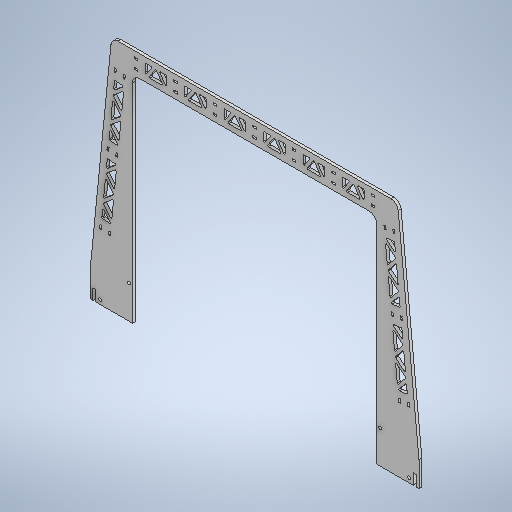
# Autodesk Inventor part: GateBrigeSideLessMaterial
Saved by Autodesk Inventor 2025.1 (Build 291241000, 241)
## iProperties
Created: 2025-03-30
Part Number: GateBrigeSideLessMaterial
Material: Všeobecné
Document SubType Name: Modeling
Designer: 42060
Density: 1 g/cm^3
Appearance: Výchozí
Author: 42060
Autodesk Inventor part; units mm, degrees
ref_plane "YZ Plane" through (0, 0, 0) normal (1, 0, 0) x (0, 1, 0)
ref_plane "XZ Plane" through (0, 0, 0) normal (0, 1, 0) x (-1, 0, 0)
ref_plane "XY Plane" through (0, 0, 0) normal (0, 0, 1) x (1, 0, 0)
sketch "Náčrt1" plane through (0, 0, 0) normal (0, 0, 1) x (1, 0, 0)
  line L0 (0, 0) -> (-160, 0)
  line L1 (-170, -10) -> (-170, -300)
  line L2 (-229, -300) -> (-229, -265.3)
  line L3 (-190.0509, 30) -> (0, 30)
  line L4 (0, 30) -> (0, 0)
  line L5 (-203.7, -249) -> (-170, -249)
  line L6 (-170, -249) -> (-170, -299)
  line L7 (-170, -299) -> (-220, -299)
  line L8 (-220, -299) -> (-220, -265.3)
  line L9 (-220, -265.3) -> (-203.7, -249)
  line L10 (-220, -299) -> (-170, -249) construction
  circle A0 centre (-215, -294) radius 2.1
  circle A1 centre (-175, -254) radius 2.1
  arc A2 (-160, 0) -> (-170, -10) centre (-160, -10) ccw
  line L11 (-200, 21.0077) -> (-229, -265.3)
  arc A3 (-190.0509, 30) -> (-200, 21.0077) centre (-190.0509, 20) ccw
  line L12 (-225, -300) -> (-225, -285)
  line L13 (-225, -285) -> (-221, -285)
  line L14 (-221, -285) -> (-221, -300)
  line L15 (-170, -300) -> (-221, -300)
  line L16 (-225, -300) -> (-229, -300)
  line L17 (0, 0) -> (160, 0)
  line L18 (170, -10) -> (170, -300)
  line L19 (229, -300) -> (229, -265.3)
  line L20 (190.0509, 30) -> (0, 30)
  line L21 (203.7, -249) -> (170, -249)
  line L22 (170, -249) -> (170, -299)
  line L23 (170, -299) -> (220, -299)
  line L24 (220, -299) -> (220, -265.3)
  line L25 (220, -265.3) -> (203.7, -249)
  line L26 (220, -299) -> (170, -249) construction
  circle A4 centre (215, -294) radius 2.1
  circle A5 centre (175, -254) radius 2.1
  arc A6 (170, -10) -> (160, 0) centre (160, -10) ccw
  line L27 (200, 21.0077) -> (229, -265.3)
  arc A7 (200, 21.0077) -> (190.0509, 30) centre (190.0509, 20) ccw
  line L28 (225, -300) -> (225, -285)
  line L29 (225, -285) -> (221, -285)
  line L30 (221, -285) -> (221, -300)
  line L31 (170, -300) -> (221, -300)
  line L32 (225, -300) -> (229, -300)
  line L33 (-36.6095, 9.0611) -> (-28.3278, 21.2788)
  line L34 (-26.6722, 21.2788) -> (-18.3905, 9.0611)
  line L35 (-19.2183, 7.5) -> (-35.7817, 7.5)
  line L36 (-21.6095, 20.9389) -> (-14.3278, 10.1964)
  line L37 (-12.5, 10.7575) -> (-12.5, 21.5)
  line L38 (-13.5, 22.5) -> (-20.7817, 22.5)
  line L39 (-33.3905, 20.9389) -> (-40.6722, 10.1964)
  line L40 (-42.5, 10.7575) -> (-42.5, 21.5)
  line L41 (-41.5, 22.5) -> (-34.2183, 22.5)
  line L42 (-55, 15) -> (0, 15) construction
  arc A8 (-41.5, 22.5) -> (-42.5, 21.5) centre (-41.5, 21.5) ccw
  arc A9 (-33.3905, 20.9389) -> (-34.2183, 22.5) centre (-34.2183, 21.5) ccw
  arc A10 (-42.5, 10.7575) -> (-40.6722, 10.1964) centre (-41.5, 10.7575) ccw
  arc A11 (-36.6095, 9.0611) -> (-35.7817, 7.5) centre (-35.7817, 8.5) ccw
  arc A12 (-19.2183, 7.5) -> (-18.3905, 9.0611) centre (-19.2183, 8.5) ccw
  arc A13 (-26.6722, 21.2788) -> (-28.3278, 21.2788) centre (-27.5, 20.7178) ccw
  arc A14 (-20.7817, 22.5) -> (-21.6095, 20.9389) centre (-20.7817, 21.5) ccw
  arc A15 (-12.5, 21.5) -> (-13.5, 22.5) centre (-13.5, 21.5) ccw
  arc A16 (-14.3278, 10.1964) -> (-12.5, 10.7575) centre (-13.5, 10.7575) ccw
  arc A17 (-81.6722, 21.2788) -> (-83.3278, 21.2788) centre (-82.5, 20.7178) ccw
  line L43 (-91.6095, 9.0611) -> (-83.3278, 21.2788)
  line L44 (-68.5, 22.5) -> (-75.7817, 22.5)
  arc A18 (-67.5, 21.5) -> (-68.5, 22.5) centre (-68.5, 21.5) ccw
  line L45 (-81.6722, 21.2788) -> (-73.3905, 9.0611)
  arc A19 (-74.2183, 7.5) -> (-73.3905, 9.0611) centre (-74.2183, 8.5) ccw
  line L46 (-76.6095, 20.9389) -> (-69.3278, 10.1964)
  line L47 (-74.2183, 7.5) -> (-90.7817, 7.5)
  arc A20 (-69.3278, 10.1964) -> (-67.5, 10.7575) centre (-68.5, 10.7575) ccw
  line L48 (-110, 15) -> (-55, 15) construction
  arc A21 (-96.5, 22.5) -> (-97.5, 21.5) centre (-96.5, 21.5) ccw
  arc A22 (-97.5, 10.7575) -> (-95.6722, 10.1964) centre (-96.5, 10.7575) ccw
  arc A23 (-91.6095, 9.0611) -> (-90.7817, 7.5) centre (-90.7817, 8.5) ccw
  arc A24 (-88.3905, 20.9389) -> (-89.2183, 22.5) centre (-89.2183, 21.5) ccw
  line L49 (-67.5, 10.7575) -> (-67.5, 21.5)
  arc A25 (-75.7817, 22.5) -> (-76.6095, 20.9389) centre (-75.7817, 21.5) ccw
  line L50 (-96.5, 22.5) -> (-89.2183, 22.5)
  line L51 (-88.3905, 20.9389) -> (-95.6722, 10.1964)
  line L52 (-97.5, 10.7575) -> (-97.5, 21.5)
  arc A26 (-136.6722, 21.2788) -> (-138.3278, 21.2788) centre (-137.5, 20.7178) ccw
  line L53 (-146.6095, 9.0611) -> (-138.3278, 21.2788)
  line L54 (-123.5, 22.5) -> (-130.7817, 22.5)
  arc A27 (-122.5, 21.5) -> (-123.5, 22.5) centre (-123.5, 21.5) ccw
  line L55 (-136.6722, 21.2788) -> (-128.3905, 9.0611)
  arc A28 (-129.2183, 7.5) -> (-128.3905, 9.0611) centre (-129.2183, 8.5) ccw
  line L56 (-131.6095, 20.9389) -> (-124.3278, 10.1964)
  line L57 (-129.2183, 7.5) -> (-145.7817, 7.5)
  arc A29 (-124.3278, 10.1964) -> (-122.5, 10.7575) centre (-123.5, 10.7575) ccw
  line L58 (-165, 15) -> (-110, 15) construction
  arc A30 (-151.5, 22.5) -> (-152.5, 21.5) centre (-151.5, 21.5) ccw
  arc A31 (-152.5, 10.7575) -> (-150.6722, 10.1964) centre (-151.5, 10.7575) ccw
  arc A32 (-146.6095, 9.0611) -> (-145.7817, 7.5) centre (-145.7817, 8.5) ccw
  arc A33 (-143.3905, 20.9389) -> (-144.2183, 22.5) centre (-144.2183, 21.5) ccw
  line L59 (-122.5, 10.7575) -> (-122.5, 21.5)
  arc A34 (-130.7817, 22.5) -> (-131.6095, 20.9389) centre (-130.7817, 21.5) ccw
  line L60 (-151.5, 22.5) -> (-144.2183, 22.5)
  line L61 (-143.3905, 20.9389) -> (-150.6722, 10.1964)
  line L62 (-152.5, 10.7575) -> (-152.5, 21.5)
  line L63 (-194.0109, -19.4488) -> (-184.1326, -20.4494)
  line L64 (-183.6011, -22.2191) -> (-194.48, -31.0969)
  line L65 (-196.1072, -30.2213) -> (-195.1066, -20.3429)
  line L66 (-182.544, -28.7227) -> (-184.7467, -50.4692)
  line L67 (-186.5164, -51.0007) -> (-196.2883, -39.0261)
  line L68 (-196.1458, -37.6191) -> (-184.1711, -27.8471)
  line L69 (-195.9642, -45.7498) -> (-186.1923, -57.7245)
  line L70 (-186.3348, -59.1315) -> (-198.3095, -68.9034)
  line L71 (-199.9366, -68.0279) -> (-197.7339, -46.2813)
  line L72 (-188.0006, -65.6537) -> (-199.9752, -75.4256)
  line L73 (-200.1177, -76.8326) -> (-190.3458, -88.8073)
  line L74 (-188.5761, -88.2758) -> (-186.3734, -66.5292)
  line L75 (-199.7937, -83.5564) -> (-190.9158, -94.4353)
  line L76 (-191.7914, -96.0625) -> (-201.6698, -95.0619)
  line L77 (-202.5639, -93.9662) -> (-201.5633, -84.0878)
  line L78 (-189.0718, -19.9491) -> (-188.1144, -10.4975) construction
  arc A35 (-194.0109, -19.4488) -> (-195.1066, -20.3429) centre (-194.1117, -20.4437) ccw
  arc A36 (-183.6011, -22.2191) -> (-184.1326, -20.4494) centre (-184.2333, -21.4443) ccw
  arc A37 (-196.1072, -30.2213) -> (-194.48, -31.0969) centre (-195.1123, -30.3221) ccw
  arc A38 (-196.1458, -37.6191) -> (-196.2883, -39.0261) centre (-195.5135, -38.3938) ccw
  arc A39 (-186.5164, -51.0007) -> (-184.7467, -50.4692) centre (-185.7416, -50.3685) ccw
  arc A40 (-182.544, -28.7227) -> (-184.1711, -27.8471) centre (-183.5389, -28.6219) ccw
  arc A41 (-195.9642, -45.7498) -> (-197.7339, -46.2813) centre (-196.739, -46.3821) ccw
  arc A42 (-186.3348, -59.1315) -> (-186.1923, -57.7245) centre (-186.9671, -58.3567) ccw
  arc A43 (-199.9366, -68.0279) -> (-198.3095, -68.9034) centre (-198.9417, -68.1287) ccw
  arc A44 (-199.9752, -75.4256) -> (-200.1177, -76.8326) centre (-199.343, -76.2004) ccw
  arc A45 (-190.3458, -88.8073) -> (-188.5761, -88.2758) centre (-189.571, -88.175) ccw
  arc A46 (-186.3734, -66.5292) -> (-188.0006, -65.6537) centre (-187.3683, -66.4284) ccw
  arc A47 (-199.7937, -83.5564) -> (-201.5633, -84.0878) centre (-200.5684, -84.1886) ccw
  arc A48 (-202.5639, -93.9662) -> (-201.6698, -95.0619) centre (-201.569, -94.067) ccw
  arc A49 (-191.7914, -96.0625) -> (-190.9158, -94.4353) centre (-191.6906, -95.0676) ccw
  arc A50 (-212.6413, -193.4572) -> (-211.7472, -194.5528) centre (-211.6464, -193.5579) ccw
  line L79 (-201.8688, -195.5534) -> (-211.7472, -194.5528)
  arc A51 (-201.8688, -195.5534) -> (-200.9932, -193.9263) centre (-201.768, -194.5585) ccw
  arc A52 (-200.4232, -188.2982) -> (-198.6535, -187.7667) centre (-199.6484, -187.666) ccw
  line L80 (-209.871, -183.0473) -> (-200.9932, -193.9263)
  line L81 (-212.6413, -193.4572) -> (-211.6407, -183.5788)
  arc A53 (-209.871, -183.0473) -> (-211.6407, -183.5788) centre (-210.6458, -183.6796) ccw
  line L82 (-198.078, -165.1446) -> (-210.0526, -174.9165)
  line L83 (-210.1951, -176.3236) -> (-200.4232, -188.2982)
  line L84 (-198.6535, -187.7667) -> (-196.4508, -166.0201)
  arc A54 (-210.0526, -174.9165) -> (-210.1951, -176.3236) centre (-209.4204, -175.6913) ccw
  arc A55 (-210.014, -167.5188) -> (-208.3869, -168.3944) centre (-209.0191, -167.6196) ccw
  arc A56 (-196.4508, -166.0201) -> (-198.078, -165.1446) centre (-197.4457, -165.9194) ccw
  line L85 (-206.0416, -145.2407) -> (-196.2697, -157.2154)
  arc A57 (-196.4122, -158.6224) -> (-196.2697, -157.2154) centre (-197.0445, -157.8476) ccw
  line L86 (-210.014, -167.5188) -> (-207.8113, -145.7722)
  line L87 (-196.4122, -158.6224) -> (-208.3869, -168.3944)
  arc A58 (-196.5938, -150.4917) -> (-194.8241, -149.9602) centre (-195.819, -149.8594) ccw
  arc A59 (-206.0416, -145.2407) -> (-207.8113, -145.7722) centre (-206.8164, -145.873) ccw
  line L88 (-196.5938, -150.4917) -> (-206.3657, -138.517)
  arc A60 (-206.2232, -137.11) -> (-206.3657, -138.517) centre (-205.5909, -137.8848) ccw
  arc A61 (-206.1846, -129.7123) -> (-204.5574, -130.5878) centre (-205.1897, -129.813) ccw
  line L89 (-192.6214, -128.2136) -> (-194.8241, -149.9602)
  line L90 (-206.2232, -137.11) -> (-194.2485, -127.338)
  arc A62 (-192.6214, -128.2136) -> (-194.2485, -127.338) centre (-193.6163, -128.1128) ccw
  arc A63 (-193.6785, -121.71) -> (-194.21, -119.9403) centre (-194.3107, -120.9352) ccw
  line L91 (-199.1491, -119.44) -> (-198.1918, -109.9884) construction
  line L92 (-204.0883, -118.9397) -> (-194.21, -119.9403)
  arc A64 (-204.0883, -118.9397) -> (-205.184, -119.8339) centre (-204.1891, -119.9346) ccw
  line L93 (-193.6785, -121.71) -> (-204.5574, -130.5878)
  line L94 (-206.1846, -129.7123) -> (-205.184, -119.8339)
  line L95 (36.6095, 9.0611) -> (28.3278, 21.2788)
  line L96 (26.6722, 21.2788) -> (18.3905, 9.0611)
  line L97 (19.2183, 7.5) -> (35.7817, 7.5)
  line L98 (21.6095, 20.9389) -> (14.3278, 10.1964)
  line L99 (12.5, 10.7575) -> (12.5, 21.5)
  line L100 (13.5, 22.5) -> (20.7817, 22.5)
  line L101 (33.3905, 20.9389) -> (40.6722, 10.1964)
  line L102 (42.5, 10.7575) -> (42.5, 21.5)
  line L103 (41.5, 22.5) -> (34.2183, 22.5)
  line L104 (55, 15) -> (0, 15) construction
  arc A65 (42.5, 21.5) -> (41.5, 22.5) centre (41.5, 21.5) ccw
  arc A66 (34.2183, 22.5) -> (33.3905, 20.9389) centre (34.2183, 21.5) ccw
  arc A67 (40.6722, 10.1964) -> (42.5, 10.7575) centre (41.5, 10.7575) ccw
  arc A68 (35.7817, 7.5) -> (36.6095, 9.0611) centre (35.7817, 8.5) ccw
  arc A69 (18.3905, 9.0611) -> (19.2183, 7.5) centre (19.2183, 8.5) ccw
  arc A70 (28.3278, 21.2788) -> (26.6722, 21.2788) centre (27.5, 20.7178) ccw
  arc A71 (21.6095, 20.9389) -> (20.7817, 22.5) centre (20.7817, 21.5) ccw
  arc A72 (13.5, 22.5) -> (12.5, 21.5) centre (13.5, 21.5) ccw
  arc A73 (12.5, 10.7575) -> (14.3278, 10.1964) centre (13.5, 10.7575) ccw
  line L105 (67.5, 10.7575) -> (67.5, 21.5)
  line L106 (96.5, 22.5) -> (89.2183, 22.5)
  arc A74 (97.5, 21.5) -> (96.5, 22.5) centre (96.5, 21.5) ccw
  line L107 (97.5, 10.7575) -> (97.5, 21.5)
  arc A75 (95.6722, 10.1964) -> (97.5, 10.7575) centre (96.5, 10.7575) ccw
  arc A76 (67.5, 10.7575) -> (69.3278, 10.1964) centre (68.5, 10.7575) ccw
  arc A77 (68.5, 22.5) -> (67.5, 21.5) centre (68.5, 21.5) ccw
  arc A78 (89.2183, 22.5) -> (88.3905, 20.9389) centre (89.2183, 21.5) ccw
  arc A79 (83.3278, 21.2788) -> (81.6722, 21.2788) centre (82.5, 20.7178) ccw
  line L108 (88.3905, 20.9389) -> (95.6722, 10.1964)
  line L109 (91.6095, 9.0611) -> (83.3278, 21.2788)
  arc A80 (76.6095, 20.9389) -> (75.7817, 22.5) centre (75.7817, 21.5) ccw
  arc A81 (90.7817, 7.5) -> (91.6095, 9.0611) centre (90.7817, 8.5) ccw
  line L110 (110, 15) -> (55, 15) construction
  line L111 (68.5, 22.5) -> (75.7817, 22.5)
  line L112 (76.6095, 20.9389) -> (69.3278, 10.1964)
  line L113 (81.6722, 21.2788) -> (73.3905, 9.0611)
  arc A82 (73.3905, 9.0611) -> (74.2183, 7.5) centre (74.2183, 8.5) ccw
  line L114 (74.2183, 7.5) -> (90.7817, 7.5)
  line L115 (122.5, 10.7575) -> (122.5, 21.5)
  line L116 (151.5, 22.5) -> (144.2183, 22.5)
  arc A83 (152.5, 21.5) -> (151.5, 22.5) centre (151.5, 21.5) ccw
  line L117 (152.5, 10.7575) -> (152.5, 21.5)
  arc A84 (150.6722, 10.1964) -> (152.5, 10.7575) centre (151.5, 10.7575) ccw
  arc A85 (122.5, 10.7575) -> (124.3278, 10.1964) centre (123.5, 10.7575) ccw
  arc A86 (123.5, 22.5) -> (122.5, 21.5) centre (123.5, 21.5) ccw
  arc A87 (144.2183, 22.5) -> (143.3905, 20.9389) centre (144.2183, 21.5) ccw
  arc A88 (138.3278, 21.2788) -> (136.6722, 21.2788) centre (137.5, 20.7178) ccw
  line L118 (143.3905, 20.9389) -> (150.6722, 10.1964)
  line L119 (146.6095, 9.0611) -> (138.3278, 21.2788)
  arc A89 (131.6095, 20.9389) -> (130.7817, 22.5) centre (130.7817, 21.5) ccw
  arc A90 (145.7817, 7.5) -> (146.6095, 9.0611) centre (145.7817, 8.5) ccw
  line L120 (165, 15) -> (110, 15) construction
  line L121 (123.5, 22.5) -> (130.7817, 22.5)
  line L122 (131.6095, 20.9389) -> (124.3278, 10.1964)
  line L123 (136.6722, 21.2788) -> (128.3905, 9.0611)
  arc A91 (128.3905, 9.0611) -> (129.2183, 7.5) centre (129.2183, 8.5) ccw
  line L124 (129.2183, 7.5) -> (145.7817, 7.5)
  line L125 (194.0109, -19.4488) -> (184.1326, -20.4494)
  line L126 (183.6011, -22.2191) -> (194.48, -31.0969)
  line L127 (196.1072, -30.2213) -> (195.1066, -20.3429)
  line L128 (182.544, -28.7227) -> (184.7467, -50.4692)
  line L129 (186.5164, -51.0007) -> (196.2883, -39.0261)
  line L130 (196.1458, -37.6191) -> (184.1711, -27.8471)
  line L131 (195.9642, -45.7498) -> (186.1923, -57.7245)
  line L132 (186.3348, -59.1315) -> (198.3095, -68.9034)
  line L133 (199.9366, -68.0279) -> (197.7339, -46.2813)
  line L134 (188.0006, -65.6537) -> (199.9752, -75.4256)
  line L135 (200.1177, -76.8326) -> (190.3458, -88.8073)
  line L136 (188.5761, -88.2758) -> (186.3734, -66.5292)
  line L137 (199.7937, -83.5564) -> (190.9158, -94.4353)
  line L138 (191.7914, -96.0625) -> (201.6698, -95.0619)
  line L139 (202.5639, -93.9662) -> (201.5633, -84.0878)
  arc A92 (195.1066, -20.3429) -> (194.0109, -19.4488) centre (194.1117, -20.4437) ccw
  arc A93 (184.1326, -20.4494) -> (183.6011, -22.2191) centre (184.2333, -21.4443) ccw
  arc A94 (194.48, -31.0969) -> (196.1072, -30.2213) centre (195.1123, -30.3221) ccw
  arc A95 (196.2883, -39.0261) -> (196.1458, -37.6191) centre (195.5135, -38.3938) ccw
  arc A96 (184.7467, -50.4692) -> (186.5164, -51.0007) centre (185.7416, -50.3685) ccw
  arc A97 (184.1711, -27.8471) -> (182.544, -28.7227) centre (183.5389, -28.6219) ccw
  arc A98 (197.7339, -46.2813) -> (195.9642, -45.7498) centre (196.739, -46.3821) ccw
  arc A99 (186.1923, -57.7245) -> (186.3348, -59.1315) centre (186.9671, -58.3567) ccw
  arc A100 (198.3095, -68.9034) -> (199.9366, -68.0279) centre (198.9417, -68.1287) ccw
  arc A101 (200.1177, -76.8326) -> (199.9752, -75.4256) centre (199.343, -76.2004) ccw
  arc A102 (188.5761, -88.2758) -> (190.3458, -88.8073) centre (189.571, -88.175) ccw
  arc A103 (188.0006, -65.6537) -> (186.3734, -66.5292) centre (187.3683, -66.4284) ccw
  arc A104 (201.5633, -84.0878) -> (199.7937, -83.5564) centre (200.5684, -84.1886) ccw
  arc A105 (201.6698, -95.0619) -> (202.5639, -93.9662) centre (201.569, -94.067) ccw
  arc A106 (190.9158, -94.4353) -> (191.7914, -96.0625) centre (191.6906, -95.0676) ccw
  arc A107 (194.21, -119.9403) -> (193.6785, -121.71) centre (194.3107, -120.9352) ccw
  arc A108 (194.2485, -127.338) -> (192.6214, -128.2136) centre (193.6163, -128.1128) ccw
  line L140 (204.0883, -118.9397) -> (194.21, -119.9403)
  line L141 (193.6785, -121.71) -> (204.5574, -130.5878)
  line L142 (206.1846, -129.7123) -> (205.184, -119.8339)
  line L143 (206.2232, -137.11) -> (194.2485, -127.338)
  arc A109 (205.184, -119.8339) -> (204.0883, -118.9397) centre (204.1891, -119.9346) ccw
  arc A110 (204.5574, -130.5878) -> (206.1846, -129.7123) centre (205.1897, -129.813) ccw
  line L144 (192.6214, -128.2136) -> (194.8241, -149.9602)
  arc A111 (207.8113, -145.7722) -> (206.0416, -145.2407) centre (206.8164, -145.873) ccw
  line L145 (196.5938, -150.4917) -> (206.3657, -138.517)
  arc A112 (206.3657, -138.517) -> (206.2232, -137.11) centre (205.5909, -137.8848) ccw
  arc A113 (194.8241, -149.9602) -> (196.5938, -150.4917) centre (195.819, -149.8594) ccw
  line L146 (206.0416, -145.2407) -> (196.2697, -157.2154)
  arc A114 (196.2697, -157.2154) -> (196.4122, -158.6224) centre (197.0445, -157.8476) ccw
  arc A115 (198.078, -165.1446) -> (196.4508, -166.0201) centre (197.4457, -165.9194) ccw
  line L147 (196.4122, -158.6224) -> (208.3869, -168.3944)
  arc A116 (208.3869, -168.3944) -> (210.014, -167.5188) centre (209.0191, -167.6196) ccw
  line L148 (210.014, -167.5188) -> (207.8113, -145.7722)
  arc A117 (200.9932, -193.9263) -> (201.8688, -195.5534) centre (201.768, -194.5585) ccw
  arc A118 (211.7472, -194.5528) -> (212.6413, -193.4572) centre (211.6464, -193.5579) ccw
  arc A119 (198.6535, -187.7667) -> (200.4232, -188.2982) centre (199.6484, -187.666) ccw
  line L149 (212.6413, -193.4572) -> (211.6407, -183.5788)
  line L150 (209.871, -183.0473) -> (200.9932, -193.9263)
  arc A120 (211.6407, -183.5788) -> (209.871, -183.0473) centre (210.6458, -183.6796) ccw
  line L151 (210.1951, -176.3236) -> (200.4232, -188.2982)
  arc A121 (210.1951, -176.3236) -> (210.0526, -174.9165) centre (209.4204, -175.6913) ccw
  line L152 (198.6535, -187.7667) -> (196.4508, -166.0201)
  line L153 (198.078, -165.1446) -> (210.0526, -174.9165)
  line L154 (201.8688, -195.5534) -> (211.7472, -194.5528)
  line L155 (-2.5, 10) -> (2.5, 10)
  line L156 (2.5, 10) -> (2.5, 7.5)
  line L157 (2.5, 7.5) -> (-2.5, 7.5)
  line L158 (-2.5, 7.5) -> (-2.5, 10)
  line L159 (-2.5, 22.5) -> (2.5, 22.5)
  line L160 (2.5, 22.5) -> (2.5, 20)
  line L161 (2.5, 20) -> (-2.5, 20)
  line L162 (-2.5, 20) -> (-2.5, 22.5)
  line L163 (0, 20) -> (0, 10) construction
  line L164 (-42.5, 10.7575) -> (-42.5, 7.5) construction
  line L165 (-42.5, 7.5) -> (-40.6722, 10.1964) construction
  line L166 (-27.5, 22.5) -> (-27.5, 7.5) construction
  line L167 (-52.5, 10) -> (-52.5, 7.5)
  line L168 (-57.5, 10) -> (-52.5, 10)
  line L169 (-52.5, 7.5) -> (-57.5, 7.5)
  line L170 (-57.5, 7.5) -> (-57.5, 10)
  line L171 (-57.5, 22.5) -> (-52.5, 22.5)
  line L172 (-52.5, 20) -> (-57.5, 20)
  line L173 (-57.5, 20) -> (-57.5, 22.5)
  line L174 (-52.5, 22.5) -> (-52.5, 20)
  line L175 (-107.5, 10) -> (-107.5, 7.5)
  line L176 (-112.5, 10) -> (-107.5, 10)
  line L177 (-107.5, 7.5) -> (-112.5, 7.5)
  line L178 (-112.5, 7.5) -> (-112.5, 10)
  line L179 (-112.5, 22.5) -> (-107.5, 22.5)
  line L180 (-107.5, 20) -> (-112.5, 20)
  line L181 (-112.5, 20) -> (-112.5, 22.5)
  line L182 (-107.5, 22.5) -> (-107.5, 20)
  line L183 (-162.5, 10) -> (-162.5, 7.5)
  line L184 (-167.5, 10) -> (-162.5, 10)
  line L185 (-162.5, 7.5) -> (-167.5, 7.5)
  line L186 (-167.5, 7.5) -> (-167.5, 10)
  line L187 (-167.5, 22.5) -> (-162.5, 22.5)
  line L188 (-162.5, 20) -> (-167.5, 20)
  line L189 (-167.5, 20) -> (-167.5, 22.5)
  line L190 (-162.5, 22.5) -> (-162.5, 20)
  line L191 (52.5, 20) -> (52.5, 22.5)
  line L192 (57.5, 20) -> (52.5, 20)
  line L193 (57.5, 22.5) -> (57.5, 20)
  line L194 (52.5, 22.5) -> (57.5, 22.5)
  line L195 (57.5, 10) -> (57.5, 7.5)
  line L196 (52.5, 10) -> (57.5, 10)
  line L197 (57.5, 7.5) -> (52.5, 7.5)
  line L198 (52.5, 7.5) -> (52.5, 10)
  line L199 (107.5, 20) -> (107.5, 22.5)
  line L200 (112.5, 20) -> (107.5, 20)
  line L201 (112.5, 22.5) -> (112.5, 20)
  line L202 (107.5, 22.5) -> (112.5, 22.5)
  line L203 (112.5, 10) -> (112.5, 7.5)
  line L204 (107.5, 10) -> (112.5, 10)
  line L205 (112.5, 7.5) -> (107.5, 7.5)
  line L206 (107.5, 7.5) -> (107.5, 10)
  line L207 (162.5, 20) -> (162.5, 22.5)
  line L208 (167.5, 20) -> (162.5, 20)
  line L209 (167.5, 22.5) -> (167.5, 20)
  line L210 (162.5, 22.5) -> (167.5, 22.5)
  line L211 (167.5, 10) -> (167.5, 7.5)
  line L212 (162.5, 10) -> (167.5, 10)
  line L213 (167.5, 7.5) -> (162.5, 7.5)
  line L214 (162.5, 7.5) -> (162.5, 10)
  line L215 (-195.0723, -4.7671) -> (-192.5851, -5.019)
  line L216 (-192.5851, -5.019) -> (-193.0889, -9.9936)
  line L217 (-193.0889, -9.9936) -> (-195.5762, -9.7416)
  line L218 (-195.5762, -9.7416) -> (-195.0723, -4.7671)
  line L219 (-182.636, -6.0268) -> (-180.1487, -6.2787)
  line L220 (-180.1487, -6.2787) -> (-180.6526, -11.2533)
  line L221 (-180.6526, -11.2533) -> (-183.1399, -11.0013)
  line L222 (-183.1399, -11.0013) -> (-182.636, -6.0268)
  line L223 (-193.0889, -9.9936) -> (-183.1399, -11.0013) construction
  line L224 (-205.6536, -109.2326) -> (-205.1497, -104.258)
  line L225 (-202.6625, -104.51) -> (-203.1663, -109.4845)
  line L226 (-203.1663, -109.4845) -> (-205.6536, -109.2326)
  line L227 (-205.1497, -104.258) -> (-202.6625, -104.51)
  line L228 (-193.2172, -110.4923) -> (-192.7134, -105.5177)
  line L229 (-190.73, -110.7442) -> (-193.2172, -110.4923)
  line L230 (-190.2261, -105.7696) -> (-190.73, -110.7442)
  line L231 (-192.7134, -105.5177) -> (-190.2261, -105.7696)
  line L232 (-203.1663, -109.4845) -> (-193.2172, -110.4923) construction
  line L233 (-202.6625, -104.51) -> (-192.7134, -105.5177) construction
  line L234 (-197.7383, -105.5113) -> (-196.7306, -95.5622) construction
  line L235 (-215.731, -208.7235) -> (-215.2271, -203.749)
  line L236 (-212.7399, -204.0009) -> (-213.2437, -208.9755)
  line L237 (-213.2437, -208.9755) -> (-215.731, -208.7235)
  line L238 (-215.2271, -203.749) -> (-212.7399, -204.0009)
  line L239 (-203.2946, -209.9832) -> (-202.7908, -205.0086)
  line L240 (-200.8074, -210.2351) -> (-203.2946, -209.9832)
  line L241 (-200.3035, -205.2606) -> (-200.8074, -210.2351)
  line L242 (-202.7908, -205.0086) -> (-200.3035, -205.2606)
  line L243 (-213.2437, -208.9755) -> (-203.2946, -209.9832) construction
  line L244 (195.0723, -4.7671) -> (192.5851, -5.019)
  line L245 (192.5851, -5.019) -> (193.0889, -9.9936)
  line L246 (193.0889, -9.9936) -> (195.5762, -9.7416)
  line L247 (195.5762, -9.7416) -> (195.0723, -4.7671)
  line L248 (182.636, -6.0268) -> (180.1487, -6.2787)
  line L249 (180.1487, -6.2787) -> (180.6526, -11.2533)
  line L250 (180.6526, -11.2533) -> (183.1399, -11.0013)
  line L251 (183.1399, -11.0013) -> (182.636, -6.0268)
  line L252 (205.6536, -109.2326) -> (205.1497, -104.258)
  line L253 (202.6625, -104.51) -> (203.1663, -109.4845)
  line L254 (203.1663, -109.4845) -> (205.6536, -109.2326)
  line L255 (205.1497, -104.258) -> (202.6625, -104.51)
  line L256 (193.2172, -110.4923) -> (192.7134, -105.5177)
  line L257 (190.73, -110.7442) -> (193.2172, -110.4923)
  line L258 (190.2261, -105.7696) -> (190.73, -110.7442)
  line L259 (192.7134, -105.5177) -> (190.2261, -105.7696)
  line L260 (215.731, -208.7235) -> (215.2271, -203.749)
  line L261 (212.7399, -204.0009) -> (213.2437, -208.9755)
  line L262 (213.2437, -208.9755) -> (215.731, -208.7235)
  line L263 (215.2271, -203.749) -> (212.7399, -204.0009)
  line L264 (203.2946, -209.9832) -> (202.7908, -205.0086)
  line L265 (200.8074, -210.2351) -> (203.2946, -209.9832)
  line L266 (200.3035, -205.2606) -> (200.8074, -210.2351)
  line L267 (202.7908, -205.0086) -> (200.3035, -205.2606)
  line L268 (-188.1144, -10.4975) -> (-188.064, -10) construction
  point P0 (-12.5, 7.5)
  point P1 (-32.3323, 22.5)
  point P2 (-42.5, 22.5)
  point P3 (-27.5, 15)
  point P4 (-12.5, 16.1288)
  point P5 (-82.5, 22.5)
  point P6 (-82.5, 15)
  point P7 (-82.5, 7.5)
  point P8 (-87.3323, 22.5)
  point P9 (-97.5, 22.5)
  point P10 (-67.5, 7.5)
  point P11 (-67.5, 16.1288)
  point P12 (-137.5, 22.5)
  point P13 (-137.5, 15)
  point P14 (-137.5, 7.5)
  point P15 (-142.3323, 22.5)
  point P16 (-152.5, 22.5)
  point P17 (-122.5, 7.5)
  point P18 (-122.5, 16.1288)
  point P19 (-195.0059, -19.348)
  point P20 (-181.7306, -20.6927)
  point P21 (-196.3505, -32.6233)
  point P22 (-182.3007, -26.3207)
  point P23 (-184.99, -52.8712)
  point P24 (-196.9206, -38.2513)
  point P25 (-197.4906, -43.8794)
  point P26 (-185.56, -58.4992)
  point P27 (-200.1799, -70.4298)
  point P28 (-186.1301, -64.1273)
  point P29 (-200.75, -76.0579)
  point P30 (-188.8194, -90.6777)
  point P31 (-201.32, -81.6859)
  point P32 (-189.3895, -96.3058)
  point P33 (-202.6647, -94.9611)
  point P34 (-212.7421, -194.4521)
  point P35 (-199.4669, -195.7967)
  point P36 (-198.8968, -190.1687)
  point P37 (-211.3974, -181.1769)
  point P38 (-210.8274, -175.5488)
  point P39 (-210.2573, -169.9207)
  point P40 (-196.2075, -163.6182)
  point P41 (-195.6374, -157.9902)
  point P42 (-195.0674, -152.3621)
  point P43 (-207.568, -143.3703)
  point P44 (-206.998, -137.7422)
  point P45 (-206.4279, -132.1142)
  point P46 (-192.3781, -125.8117)
  point P47 (-191.808, -120.1836)
  point P48 (-205.0833, -118.839)
  point P49 (27.5, 22.5)
  point P50 (12.5, 7.5)
  point P51 (32.3323, 22.5)
  point P52 (42.5, 22.5)
  point P53 (27.5, 7.5)
  point P54 (27.5, 15)
  point P55 (12.5, 16.1288)
  point P56 (67.5, 7.5)
  point P57 (67.5, 16.1288)
  point P58 (82.5, 22.5)
  point P59 (87.3323, 22.5)
  point P60 (97.5, 22.5)
  point P61 (82.5, 15)
  point P62 (82.5, 7.5)
  point P63 (122.5, 7.5)
  point P64 (122.5, 16.1288)
  point P65 (137.5, 22.5)
  point P66 (142.3323, 22.5)
  point P67 (152.5, 22.5)
  point P68 (137.5, 15)
  point P69 (137.5, 7.5)
  point P70 (195.0059, -19.348)
  point P71 (181.7306, -20.6927)
  point P72 (196.3505, -32.6233)
  point P73 (182.3007, -26.3207)
  point P74 (184.99, -52.8712)
  point P75 (196.9206, -38.2513)
  point P76 (197.4906, -43.8794)
  point P77 (185.56, -58.4992)
  point P78 (200.1799, -70.4298)
  point P79 (186.1301, -64.1273)
  point P80 (200.75, -76.0579)
  point P81 (188.8194, -90.6777)
  point P82 (201.32, -81.6859)
  point P83 (189.3895, -96.3058)
  point P84 (202.6647, -94.9611)
  point P85 (189.0718, -19.9491)
  point P86 (191.808, -120.1836)
  point P87 (192.3781, -125.8117)
  point P88 (199.1491, -119.44)
  point P89 (205.0833, -118.839)
  point P90 (206.4279, -132.1142)
  point P91 (206.998, -137.7422)
  point P92 (195.0674, -152.3621)
  point P93 (207.568, -143.3703)
  point P94 (195.6374, -157.9902)
  point P95 (196.2075, -163.6182)
  point P96 (210.2573, -169.9207)
  point P97 (212.7421, -194.4521)
  point P98 (199.4669, -195.7967)
  point P99 (198.8968, -190.1687)
  point P100 (210.8274, -175.5488)
  point P101 (211.3974, -181.1769)
  point P102 (0, 15)
  point P103 (-27.5, 15)
  point P104 (-55, 10)
  point P105 (-55, 20)
  point P106 (-110, 10)
  point P107 (-110, 20)
  point P108 (-165, 10)
  point P109 (-165, 20)
  point P110 (55, 20)
  point P111 (55, 10)
  point P112 (110, 20)
  point P113 (110, 10)
  point P114 (165, 20)
  point P115 (165, 10)
  point P116 (-198.1918, -109.9884)
  point P117 (-208.2692, -209.4793)
  point P118 (-197.6879, -105.0138)
  dimension "d0" = 50
  dimension "d1" = 50
  dimension "d3" = 33.7
  dimension "d4" = 45
  dimension "d5" = 0
  dimension "d6" = 4.2
  dimension "d7" = 5
  dimension "d8" = 5
  dimension "d10" = 170
  dimension "d12" = 30
  dimension "d14" = 10
  dimension "d16" = 15
  dimension "d17" = 1
  dimension "d18" = 4
  dimension "d19" = 1
  dimension "d20" = 4
  dimension "d21" = 300
  dimension "d22" = 30
  dimension "d46" = 4
  dimension "d47" = 4
  dimension "d50" = 15
  dimension "d51" = 30
  dimension "d52" = 1
  dimension "d55" = 55
  dimension "d63" = 4
  dimension "d64" = 4
  dimension "d65" = 4
  dimension "d66" = 4
  dimension "d67" = 1
  dimension "d70" = 100
  dimension "d77" = 55
  dimension "d84" = 100
  dimension "d91" = 2.5
  dimension "d92" = 5
  dimension "d93" = 15
  dimension "d96" = 55
  dimension "d103" = 55
  dimension "d108" = 5
  dimension "d109" = 2.5
  dimension "d110" = 7.5
  dimension "d111" = 15
  dimension "d115" = 100
  dimension "d123" = 0.5
  dimension "d124" = 0.5
  dimension "d125" = 10
  dimension "d126" = 10
  constraints: 538 end point, 236 point on circle, 227 point on line, 141 symmetric about line, 122 centre point, 52 tangent, 24 equal radius, 24 perpendicular, 20 parallel, 12 midpoint, 11 collinear, 10 coincident, 10 horizontal, 5 equal length, 4 horizontal alignment, 4 vertical alignment, 2 vertical, 579 other
  measures "d0" distance of L5.end L6.end
  measures "d1" distance of L6.end L7.end
  measures "d3" distance of L5.start L5.end
  measures "d4" angle of L5 L9
  measures "d5" distance between parallel lines of L1 L6
  measures "d6" diameter of A1
  measures "d7" distance from line of L5 A1.centre
  measures "d8" distance from line of L7 A0.centre
  measures "d10" distance between parallel lines of L1 L4
  measures "d12" distance between parallel lines of L0 L3
  measures "d14" radius of A3
  measures "d16" distance between parallel lines of L16 L13
  measures "d17" distance between parallel lines of L7 L15
  measures "d18" distance between parallel lines of L14 L12
  measures "d19" distance between parallel lines of L8 L14
  measures "d20" distance between parallel lines of L12 L2
  measures "d21" distance between parallel lines of L15 L0
  measures "d22" distance from line of L11.start L1
  measures "d46" distance between parallel lines of L33 L39
  measures "d47" distance between parallel lines of L36 L34
  measures "d50" distance from line of L35 L166.start
  measures "d51" distance between parallel lines of L37 L40
  measures "d52" radius of A8
  measures "d55" distance of L166.start point (-82.5, 22.5)
  measures "d63" distance between parallel lines of L68 L64
  measures "d64" distance between parallel lines of L69 L67
  measures "d65" distance between parallel lines of L72 L70
  measures "d66" distance between parallel lines of L73 L75
  measures "d67" radius of A35
  measures "d70" distance of point (-202.665, -94.961) point (-212.742, -194.452)
  measures "d77" distance of point (12.5, 7.5) point (67.5, 7.5)
  measures "d84" distance of point (181.731, -20.693) point (191.808, -120.184)
  measures "d91" distance of L159.end L160.end
  measures "d92" distance of L159.start L159.end
  measures "d93" distance between parallel lines of L157 L159
  measures "d96" distance of L155.end L167.start
  measures "d103" distance of L159.start L191.end
  measures "d108" distance of L217.end L215.start
  measures "d109" distance of L215.start L215.end
  measures "d110" distance between parallel lines of L11 L218
  measures "d111" distance between parallel lines of L220 L218
  measures "d115" distance of L217.end L224.start
  measures "d123" distance of L268.start L268.end
  measures "d124" distance from line of L234.start L233
  measures "d125" distance of L78.start L268.end
  measures "d126" distance of L234.start L234.end
extrude "Vysunutí1" add sketch "Náčrt1" along normal blind 4 contours L0 A2 L1 L5 L9 L8 L7 L15 L14 L13 L12 L16 L2 L11 A3 L3 L4 L159 L162 L161 L155 L158 L157 | L4 L157 L156 L155 L161 L160 L159 L20 A7 L27 L19 L32 L28 L29 L30 L31 L18 L23 L24 L25 L21 A6 L17 | L1 L7 L8 L9 L5 | L21 L25 L24 L23 L18
equation "\"d44\" = d18"
